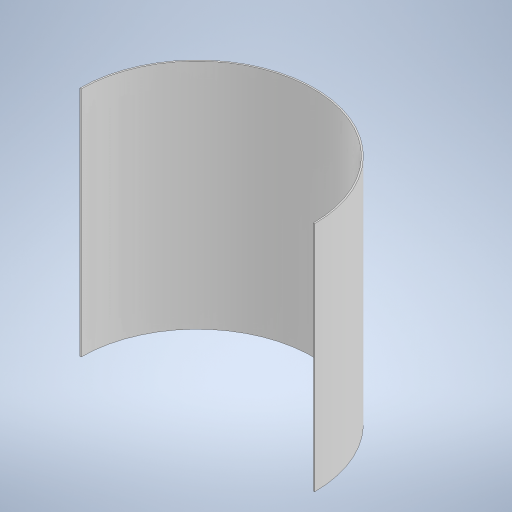
# Autodesk Inventor part: Aspa
Saved by Autodesk Inventor 2024 (Build 280153000, 153)
## iProperties
Created: 2024-04-25
Part Number: Aspa
Material: Genérico
Document SubType Name: Modeling
Designer: alexa
Density: 1 g/cm^3
Appearance: Valor por defecto
Author: alexa
Autodesk Inventor part; units mm, degrees
ref_plane "YZ Plane" through (0, 0, 0) normal (1, 0, 0) x (0, 1, 0)
ref_plane "XZ Plane" through (0, 0, 0) normal (0, 1, 0) x (-1, 0, 0)
ref_plane "XY Plane" through (0, 0, 0) normal (0, 0, 1) x (1, 0, 0)
sketch "Sketch2" plane through (0, 0, 0) normal (1, 0, 0) x (0, 1, 0)
  line L0 (0, 0) -> (121.8561, 0)
  line L1 (3, -250) -> (497, -250)
  line L2 (500, -250) -> (500, -253)
  line L3 (500, -253) -> (0, -253)
  line L4 (0, -253) -> (0, -250)
  line L5 (500, 0) -> (497, 0)
  line L6 (3, -250) -> (0, -250)
  line L7 (497, -250) -> (500, -250)
  point P0 (3, 0)
  dimension "d7" = 500
  constraints: 16 end point, 5 horizontal, 2 parallel, 1 perpendicular, 1 point on line
  measures "d7" distance of L2.end L3.end
revolve "Revolution1" add sketch "Sketch2" angle 180 mid plane about axis through (0, 0, 0) along (0, 1, 0)
body "Solid2"
